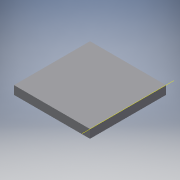
# Autodesk Inventor part: Body
Saved by Autodesk Inventor 2017.2 (Build 212223000, 223)
## iProperties
Created: 2017-02-21
Part Number: Body
Material: Generic
Document SubType Name: Modeling
Designer: prosp
Density: 1 g/cm^3
Appearance: Default
Author: prosp
Autodesk Inventor part; units mm, degrees
ref_plane "YZ Plane" through (0, 0, 0) normal (1, 0, 0) x (0, 1, 0)
ref_plane "XZ Plane" through (0, 0, 0) normal (0, 1, 0) x (-1, 0, 0)
ref_plane "XY Plane" through (0, 0, 0) normal (0, 0, 1) x (1, 0, 0)
sketch "Sketch1" plane through (0, 0, 0) normal (0, 1, 0) x (-1, 0, 0)
  line L0 (45, 35) -> (45, -35)
  line L1 (35, -45) -> (-35, -45)
  line L2 (-45, -35) -> (-45, 35)
  line L3 (-35, 45) -> (35, 45)
  line L4 (45, 45) -> (-45, -45) construction
  line L5 (45, -45) -> (-45, 45) construction
  arc A0 (35, -45) -> (45, -35) centre (35, -35) ccw
  arc A1 (-45, -35) -> (-35, -45) centre (-35, -35) ccw
  arc A2 (-35, 45) -> (-45, 35) centre (-35, 35) ccw
  arc A3 (45, 35) -> (35, 45) centre (35, 35) ccw
  point P0 (0, 0)
  dimension "d0" = 90
  dimension "d1" = 90
  dimension "d10" = 10
  constraints: 12 end point, 8 point on circle, 8 point on line, 8 tangent, 4 centre point, 3 equal radius, 2 midpoint, 2 parallel, 1 perpendicular, 1 vertical
  measures "d0" distance of L4.start L5.start
  measures "d1" distance of L5.start L4.end
  measures "d10" radius of A0
extrude "Extrusion1" add sketch "Sketch1" along normal blind 10
shell "Shell2" thickness 2 removed faces 1 at (-11.6667, 0, -15)
fillet "Fillet1" radius 5 1 edges at (-45, 10, 0)
fillet "Fillet2" [suppressed]
fillet "Fillet3" [suppressed]
fillet "Fillet4" [suppressed]
body "Solid1"
